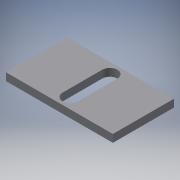
# Autodesk Inventor part: disk plate
Saved by Autodesk Inventor 2018 (Build 220112000, 112)
## iProperties
Created: 2021-03-01
Part Number: disk plate
Material: Generic
Document SubType Name: Modeling
Designer: Default
Density: 1 g/cm^3
Appearance: Default
Author: Default
Autodesk Inventor part; units mm, degrees
ref_plane "YZ Plane" through (0, 0, 0) normal (1, 0, 0) x (0, 1, 0)
ref_plane "XZ Plane" through (0, 0, 0) normal (0, 1, 0) x (-1, 0, 0)
ref_plane "XY Plane" through (0, 0, 0) normal (0, 0, 1) x (1, 0, 0)
sketch "Sketch1" plane through (0, 0, 0) normal (0, 0, 1) x (1, 0, 0)
  line L0 (0, 0) -> (350, 0)
  line L1 (350, 0) -> (350, 200)
  line L2 (350, 200) -> (0, 200)
  line L3 (0, 200) -> (0, 0)
  line L4 (175, 165) -> (175, 35) construction
  line L5 (150, 165) -> (150, 35)
  line L6 (200, 35) -> (200, 165)
  arc A0 (200, 165) -> (150, 165) centre (175, 165) ccw
  arc A1 (150, 35) -> (200, 35) centre (175, 35) ccw
  point P0 (175, 100)
  dimension "d6" = 175
  dimension "d7" = 130
  constraints: 16 end point, 4 point on circle, 4 tangent, 3 parallel, 2 centre point, 1 horizontal, 1 midpoint, 1 perpendicular, 1 vertical
  measures "d6" distance from line of L3 point (175, 100)
  measures "d7" distance of L6.start L6.end
extrude "Extrusion1" add sketch "Sketch1" along normal blind 25
body "Solid1"
